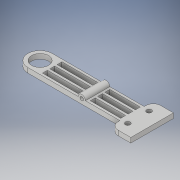
# Autodesk Inventor part: Side V4
Saved by Autodesk Inventor 2019 (Build 230136000, 136)
## iProperties
Created: 2018-11-04
Part Number: Side V4
Material: Generic
Document SubType Name: Modeling
Designer: mrhftc
Density: 1 g/cm^3
Appearance: Default
Author: mrhftc
Autodesk Inventor part; units mm, degrees
ref_plane "YZ Plane" through (0, 0, 0) normal (1, 0, 0) x (0, 1, 0)
ref_plane "XZ Plane" through (0, 0, 0) normal (0, 1, 0) x (-1, 0, 0)
ref_plane "XY Plane" through (0, 0, 0) normal (0, 0, 1) x (1, 0, 0)
sketch "Main Sketch" plane through (0, 0, 0) normal (0, 1, 0) x (-1, 0, 0)
  line L0 (-44.375, -9.3176) -> (-44.375, 9.3176)
  line L1 (-44.375, 9.3176) -> (47.625, -10) construction
  line L2 (47.625, 10) -> (-44.375, -9.3176) construction
  circle A0 centre (47.625, 0) radius 7
  arc A1 (47.625, -10) -> (47.625, 10) centre (47.625, 0) ccw
  line L3 (-27.875, 17.5) -> (-44.375, 17.5)
  line L4 (-44.375, 17.5) -> (-44.375, -17.5)
  line L5 (-44.375, -17.5) -> (-27.875, -17.5)
  line L6 (-27.875, 17.5) -> (-44.375, -17.5) construction
  line L7 (-44.375, 17.5) -> (-27.875, -17.5) construction
  line L8 (47.625, -10) -> (-27.875, -10)
  line L9 (-27.875, -17.5) -> (-27.875, -10)
  line L10 (-27.875, 10) -> (-27.875, 17.5)
  line L11 (-27.875, 10) -> (47.625, 10)
  point P0 (0, 0)
  point P1 (-36.125, 0)
  dimension "d3" = 14
  dimension "d4" = 92
  dimension "d13" = 16.5
  dimension "d14" = 35
  dimension "d15" = 0
  dimension "d18" = 20
  constraints: 24 end point, 4 parallel, 2 centre point, 2 horizontal, 2 midpoint, 2 point on circle, 2 point on line, 1 coincident, 1 perpendicular
  measures "d3" diameter of A0
  measures "d4" distance from line of L0 A0.centre
  measures "d13" distance of L4.end L5.end
  measures "d14" distance of L3.end L4.end
  measures "d15" distance between parallel lines of L0 L4
  measures "d18" distance between parallel lines of L11 L8
extrude "Main Extrusion" add sketch "Main Sketch" along normal blind 4
sketch "Screw Holes Sketch" plane through (0, 4, 0) normal (0, 1, 0) x (1, 0, 0)
  circle A0 centre (33.125, -8.75) radius 2
  line L0 (44.375, 17.5) -> (27.875, 17.5) projected
  line L1 (27.875, -17.5) -> (44.375, -17.5) projected
  line L2 (22.2664, 0) -> (52.7891, 0)
  line L3 (38.375, -27.0398) -> (38.375, 30.2346) construction
  line L4 (44.375, -17.5) -> (44.375, 17.5) projected
  line L5 (27.875, -10) -> (27.875, -17.5) projected
  circle A1 centre (33.125, 8.75) radius 2
  line L6 (38.375, 27.0398) -> (38.375, -30.2346) construction
  point P0 (0, 0)
  dimension "d21" = 4
  dimension "d22" = 35
  dimension "d23" = 6
  dimension "d24" = 5.25
  dimension "d25" = 5.25
  dimension "d26" = 10.5
  dimension "d27" = 8.75
  dimension "d28" = 17.5
  constraints: 6 end point, 3 symmetric about line, 2 centre point, 1 horizontal, 1 vertical, 1 other
  measures "d21" diameter of A0
  measures "d22" distance between parallel lines of L0 L1
  measures "d23" distance between parallel lines of L4 L3
  measures "d24" distance from line of L3 A0.centre
  measures "d25" distance from line of L5 A0.centre
  measures "d26" distance between parallel lines of L3 L5
  measures "d27" distance from line of L1 A0.centre
  measures "d28" diameter of A0.centre L2
extrude "Screw Holes Cut" cut sketch "Screw Holes Sketch" against normal through all
fillet "Smoooooooooooooooooth" radius 6 2 edges at (27.875, 2, -17.5) (27.875, 2, 17.5)
sketch "Side Axel Hole Sketch" plane through (-47.625, 0, 10) normal (0, 0, 1) x (1, 0, 0)
  line L0 (75.5, 4) -> (75.5, 0) projected
  line L1 (0, 0) -> (0, 4) projected
  line L2 (44.25, -12.0383) -> (44.25, 22.7681) construction
  line L3 (75.5, 0) -> (0, 0) projected
  line L4 (0, 4) -> (75.5, 4) projected
  circle A0 centre (44.25, 4) radius 1.5
  point P0 (47.625, 0)
  dimension "d32" = 75.5
  dimension "d33" = 44.25
  dimension "d34" = 31.25
  dimension "d35" = 4
  dimension "d41" = 3
  constraints: 2 end point, 1 centre point, 1 point on line, 1 vertical
  measures "d32" distance between parallel lines of L0 L1
  measures "d33" distance between parallel lines of L1 L2
  measures "d34" distance between parallel lines of L0 L2
  measures "d35" distance between parallel lines of L3 L4
  measures "d41" diameter of A0
extrude "Side Axel Hole Cut" cut sketch "Side Axel Hole Sketch" against normal blind 20 contours A0 L4 | L4 A0
sketch "Side Hole Extension Sketch" plane through (-47.625, 0, 10) normal (0, 0, 1) x (1, 0, 0)
  arc A0 (42.75, 4) -> (45.75, 4) centre (44.25, 4) ccw projected
  circle A1 centre (44.25, 4) radius 3
  circle A2 centre (44.25, 4) radius 1.5
  point P0 (47.625, 0)
  dimension "d44" = 6
  constraints: 2 centre point, 2 coincident, 1 concentric
  measures "d44" diameter of A1
extrude "Side Hole Extrusion" add sketch "Side Hole Extension Sketch" against normal blind 20
sketch "Body Holes Sketch" plane through (0, 4, 0) normal (0, 1, 0) x (1, 0, 0)
  line L0 (-37.625, 8) -> (-8.375, 8)
  line L1 (-8.375, 8) -> (-8.375, 4)
  line L2 (-8.375, 4) -> (-37.625, 4)
  line L3 (-37.625, 4) -> (-37.625, 8)
  line L4 (-6.375, -10) -> (-6.375, 10) projected
  circle A0 centre (-47.625, 0) radius 7 projected
  line L5 (-47.625, 7) -> (-47.625, -13.5384) construction
  line L6 (-6.375, 10) -> (-47.625, 10) projected
  line L7 (-47.625, 1) -> (-47.625, -19.5384) construction
  line L8 (-37.625, 2) -> (-8.375, 2)
  line L9 (-8.375, 2) -> (-8.375, -2)
  line L10 (-8.375, -2) -> (-37.625, -2)
  line L11 (-37.625, -2) -> (-37.625, 2)
  line L12 (-47.625, -5) -> (-47.625, -25.5384) construction
  line L13 (-37.625, -4) -> (-8.375, -4)
  line L14 (-8.375, -4) -> (-8.375, -8)
  line L15 (-8.375, -8) -> (-37.625, -8)
  line L16 (-37.625, -8) -> (-37.625, -4)
  line L17 (1.625, 8) -> (26.625, 8)
  line L18 (26.625, 8) -> (26.625, 4)
  line L19 (26.625, 4) -> (1.625, 4)
  line L20 (1.625, 4) -> (1.625, 8)
  line L21 (-0.375, 10) -> (-0.375, -10) projected
  line L22 (27.875, 10) -> (-0.375, 10) projected
  line L23 (1.625, -2) -> (1.625, 2)
  line L24 (26.625, -2) -> (1.625, -2)
  line L25 (26.625, 2) -> (26.625, -2)
  line L26 (1.625, 2) -> (26.625, 2)
  line L27 (1.625, -8) -> (1.625, -4)
  line L28 (26.625, -8) -> (1.625, -8)
  line L29 (26.625, -4) -> (26.625, -8)
  line L30 (1.625, -4) -> (26.625, -4)
  point P0 (0, 0)
  dimension "d77" = 4
  dimension "d78" = 2
  dimension "d79" = 10
  dimension "d80" = 2
  dimension "d83" = 6
  dimension "d88" = 2
  dimension "d89" = 2
  dimension "d90" = 4
  dimension "d91" = 25
  dimension "d94" = 6
  constraints: 54 end point, 4 parallel, 3 vertical, 2 horizontal, 2 perpendicular, 1 collinear, 1 vertical alignment, 38 other
  measures "d77" distance between parallel lines of L2 L0
  measures "d78" distance between parallel lines of L4 L1
  measures "d79" distance between parallel lines of L3 L5
  measures "d80" distance between parallel lines of L0 L6
  measures "d83" distance of L5.start L7.start
  measures "d88" distance between parallel lines of L20 L21
  measures "d89" distance between parallel lines of L17 L22
  measures "d90" distance between parallel lines of L19 L17
  measures "d91" distance between parallel lines of L18 L20
  measures "d94" distance of L19.end L23.start
extrude "Swiss-ified" cut sketch "Body Holes Sketch" against normal through all contours L0 L1 L2 L3 | L8 L9 L10 L11 | L13 L14 L15 L16 | L17 L18 L19 L20 | L23 L26 L25 L24 | L27 L30 L29 L28
body "Solid3"
